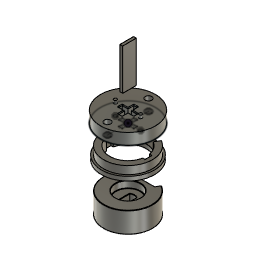
Zemismart Blinds.com Adapter (Autodesk Fusion 360 design; units mm, degrees)
Autodesk Fusion 360 part; units mm, degrees
sketch "Sketch1" plane through (0, 0, 0) normal (0, 0, 1) x (1, 0, 0) in component "Motor Driver"
  circle A0 centre (0, 0) radius 17.875
  line L0 (-9.0114, 15.4373) -> (8.9886, 15.4506)
  line L1 (-9.0114, 15.4373) -> (-5.0783, 15.4373) construction
  circle A1 centre (0, 0) radius 12.375 construction
  line L2 (-12.8986, 12.375) -> (12.8986, 12.375) construction
  line L3 (-9.0114, 15.4373) -> (-7.2434, 12.375)
  line L4 (-9.0114, 15.4373) -> (-5.4753, 15.4373) construction
  line L5 (8.9886, 15.4506) -> (7.2129, 12.375)
  line L6 (8.9886, 15.4506) -> (12.5579, 15.4506) construction
  line L7 (7.2129, 12.375) -> (-7.2434, 12.375)
  circle A2 centre (0, 0) radius 4.5
  line L8 (0, 0) -> (2.5, 0) construction
  line L9 (0, 0) -> (-2.5, 0) construction
  line L10 (-2.5, 0) -> (-2.5, 3.7417)
  line L11 (-2.5, 0) -> (-2.5, -3.7417)
  line L12 (2.5, 0) -> (2.5, -3.7417)
  line L13 (2.5, 0) -> (2.5, 3.7417)
  circle A3 centre (0, 0) radius 9.125
  dimension "d1" = 35.75
  dimension "d2" = 18
  dimension "d4" = 24.75
  dimension "d5" = 60
  dimension "d6" = 120
  dimension "d7" = 9
  dimension "d8" = 2.5
  dimension "d9" = 2.5
  dimension "d12" = 18.25
  constraint coincident A0.centre A1.centre
  constraint coincident A0 L0.start
  constraint coincident A0 L0.end
  constraint horizontal L1
  constraint coincident A0 L2.start
  constraint coincident A0 L2.end
  constraint horizontal L2
  constraint tangent A1 L2
  constraint horizontal L4
  constraint coincident L2 L3.end
  constraint horizontal L6
  constraint coincident L2 L5.end
  constraint concentric A1 A2
  constraint horizontal L8
  constraint parallel L8 L9
  constraint coincident A2 L10.end
  constraint perpendicular L9 L10
  constraint coincident A2 L11.end
  constraint perpendicular L9 L11
  constraint coincident A2 L12.end
  constraint perpendicular L8 L12
  constraint coincident A2 L13.end
  constraint perpendicular L8 L13
  constraint concentric A2 A3
  measures "d1" diameter of A0
  measures "d2" distance of L0.start L0.end
  measures "d4" diameter of A1
  measures "d5" angle of L3 L4
  measures "d6" angle of L5 L6
  measures "d7" diameter of A2
  measures "d8" distance of A0.centre L8.end
  measures "d9" distance of A0.centre L9.end
  measures "d12" diameter of A3
extrude "Extrude1" add sketch "Sketch1" along normal blind 15.25 contours A0 L3 L5 L7 | A2 L12 L13 | A2 L10 L11 | A3 makes body 1 in component "Motor Driver"
extrude "Extrude2" cut sketch "Sketch1" against normal blind 5 from surface at 15.25 contours A2 L12 L13 | A2 L10 L11 | A3 bodies 1 in component "Motor Driver"
fillet "Fillet1" radius 0.25 3 faces at (-4.7083, 0, 10.25) (9.1137, -0.4548, 11.9167) (9.0132, 10.2341, 15.25) on bodies 1 in component "Motor Driver"
fillet "Fillet2" radius 0.25 1 faces at (-0.0102, 9.75, 0) on bodies 1 in component "Motor Driver"
sketch "Sketch1 (2)" plane through (0, 0, 0) normal (0, 0, 1) x (1, 0, 0) in component "Motor Ring"
  circle A0 centre (0, 0) radius 17.875
  line L0 (-9.0114, 15.4373) -> (8.9886, 15.4506)
  line L1 (-9.0114, 15.4373) -> (-5.0783, 15.4373) construction
  circle A1 centre (0, 0) radius 2.5 construction
  line L2 (-17.6993, 2.5) -> (17.6993, 2.5) construction
  line L3 (-9.0114, 15.4373) -> (-1.5421, 2.5)
  line L4 (-9.0114, 15.4373) -> (-5.4753, 15.4373) construction
  line L5 (8.9886, 15.4506) -> (1.5115, 2.5)
  line L6 (8.9886, 15.4506) -> (12.5579, 15.4506) construction
  line L7 (1.5115, 2.5) -> (-1.5421, 2.5)
  dimension "d1_1" = 35.75
  dimension "d2_1" = 18
  dimension "d4_1" = 5
  dimension "d5_1" = 60
  dimension "d6_1" = 120
  constraint coincident A0.centre A1.centre
  constraint coincident A0 L0.start
  constraint coincident A0 L0.end
  constraint horizontal L1
  constraint coincident A0 L2.start
  constraint coincident A0 L2.end
  constraint horizontal L2
  constraint tangent A1 L2
  constraint horizontal L4
  constraint coincident L2 L3.end
  constraint horizontal L6
  constraint coincident L2 L5.end
  measures "d1_1" diameter of A0
  measures "d2_1" distance of L0.start L0.end
  measures "d4_1" diameter of A1
  measures "d5_1" angle of L3 L4
  measures "d6_1" angle of L5 L6
sketch "Ring Base" plane through (0, 0, 0) normal (0, 0, 1) x (1, 0, 0) in component "Motor Ring"
  circle A0 centre (0, 0) radius 19.375
  circle A1 centre (0, 0) radius 13.5
  line L0 (15, 2.5) -> (-15, 2.5)
  line L1 (-15, 2.5) -> (-15, -2.5)
  line L2 (-15, -2.5) -> (15, -2.5)
  line L3 (15, -2.5) -> (15, 2.5)
  line L4 (15, 2.5) -> (-15, -2.5) construction
  line L5 (-15, 2.5) -> (15, -2.5) construction
  dimension "d18" = 38.75
  dimension "d19" = 27
  dimension "d20" = 30
  dimension "d21" = 5
  constraint coincident A0.centre A1.centre
  constraint horizontal L0
  constraint perpendicular L0 L1
  constraint parallel L0 L2
  constraint parallel L1 L3
  constraint coincident L4 A0.centre
  constraint coincident L5 A0.centre
  measures "d18" diameter of A0
  measures "d19" diameter of A1
  measures "d20" distance of L1.end L2.end
  measures "d21" distance of L0.end L1.end
extrude "Extrude1'" add sketch "Ring Base" along normal blind 3 separate body makes body 2 in component "Motor Ring"
extrude "Extrude2'" add sketch "Sketch1 (2)" along normal blind 5.75 from surface at 3 contours A0 L3 L5 L7 bodies 2 in component "Motor Ring"
extrude "Extrude3" cut 1 faces at (9.3482, 0.8333, 3) along direction (0, 0, 1) blind 5.75 on bodies 2 bodies 2 in component "Motor Ring"
move_body "Move1" bodies 2 to x (1, 0, 0) y (0, 1, 0) z (0, 0, 1) at (0, 0, 25) in component "Motor Ring"
move_body "Move2" bodies 2 to x (1, 0, 0) y (0, 1, 0) z (0, 0, 1) at (0, 0, 10) in component "Motor Ring"
sketch "Sketch3" plane through (0, 0, 0) normal (0, 0, 1) x (1, 0, 0) in component "Motor Mount"
  line L0 (0, 0) -> (9.25, 0) construction
  circle A0 centre (9.25, 0) radius 1.125
  line L1 (0, 0) -> (-9.25, 0) construction
  circle A1 centre (-9.25, 0) radius 1.125
  dimension "d34_1" = 9.25
  dimension "d35_1" = 2.25
  dimension "d36_1" = 9.25
  dimension "d37_1" = 2.25
  constraint coincident L0.start L1.start
  constraint horizontal L0
  constraint coincident L0.end A0.centre
  constraint parallel L0 L1
  constraint coincident L1.end A1.centre
  measures "d34_1" distance of L0.start L0.end
  measures "d35_1" diameter of A0
  measures "d36_1" distance of L0.start L1.end
  measures "d37_1" diameter of A1
sketch "Sketch1 (3)" plane through (0, 0, 0) normal (0, 0, 1) x (1, 0, 0) in component "Motor Mount"
  circle A0 centre (0, 0) radius 20
  line L0 (0, 0) -> (0, 15) construction
  circle A1 centre (0, 15) radius 2.375
  line L1 (0, 0) -> (0, -15) construction
  circle A2 centre (0, -15) radius 2.375
  dimension "d1_2" = 40
  dimension "d2_2" = 15
  dimension "d3_1" = 4.75
  dimension "d4_2" = 15
  dimension "d5_2" = 4.75
  constraint coincident A0.centre L0.start
  constraint vertical L0
  constraint coincident L0.end A1.centre
  constraint vertical L1
  constraint coincident L1.end A2.centre
  measures "d1_2" diameter of A0
  measures "d2_2" distance of A0.centre L0.end
  measures "d3_1" diameter of A1
  measures "d4_2" distance of A0.centre L1.end
  measures "d5_2" diameter of A2
extrude "Extrude1''" add sketch "Sketch1 (3)" along normal blind 8.25 separate body makes body 3 in component "Motor Mount"
sketch "Sketch2" plane through (0, 0, 0) normal (0, 0, 1) x (1, 0, 0) in component "Motor Mount"
  line L0 (5.5, 1.25) -> (-5.5, 1.25)
  line L1 (-5.5, 1.25) -> (-5.5, -1.25)
  line L2 (-5.5, -1.25) -> (5.5, -1.25)
  line L3 (5.5, -1.25) -> (5.5, 1.25)
  line L4 (5.5, 1.25) -> (-5.5, -1.25) construction
  line L5 (-5.5, 1.25) -> (5.5, -1.25) construction
  line L6 (1.25, 5.5) -> (-1.25, 5.5)
  line L7 (-1.25, 5.5) -> (-1.25, -5.5)
  line L8 (-1.25, -5.5) -> (1.25, -5.5)
  line L9 (1.25, -5.5) -> (1.25, 5.5)
  line L10 (1.25, 5.5) -> (-1.25, -5.5) construction
  line L11 (-1.25, 5.5) -> (1.25, -5.5) construction
  dimension "d46_1" = 11
  dimension "d47_1" = 2.5
  dimension "d52_1" = 2.5
  dimension "d53_1" = 11
  constraint horizontal L0
  constraint perpendicular L0 L1
  constraint parallel L0 L2
  constraint parallel L1 L3
  constraint coincident L4 origin
  constraint coincident L5 origin
  constraint horizontal L6
  constraint perpendicular L6 L7
  constraint parallel L6 L8
  constraint parallel L7 L9
  constraint coincident L10 origin
  constraint coincident L11 origin
  measures "d46_1" distance of L1.end L2.end
  measures "d47_1" distance of L0.end L1.end
  measures "d52_1" distance of L7.end L8.end
  measures "d53_1" distance of L6.end L7.end
extrude "Extrude3'" add sketch "Sketch3" along normal blind 2.25 from surface at 8.25 bodies 3 in component "Motor Mount"
chamfer "Chamfer1" distance 0.75 angle 45 1 edges at (-2.2143, -14.1412, 0) on bodies 3 in component "Motor Mount"
chamfer "Chamfer2" distance 0.75 angle 45 1 edges at (-2.2143, 15.8588, 0) on bodies 3 in component "Motor Mount"
extrude "Extrude4" cut sketch "Sketch2" against normal blind 8 from surface at 8.25 bodies 3 in component "Motor Mount"
fillet "Fillet3" radius 0.5 6 edges at (3.375, 1.25, 8.25) (-3.375, 1.25, 8.25) (-5.5, 0, 8.25) (3.375, -1.25, 8.25) (-3.375, -1.25, 8.25) (5.5, 0, 8.25) on bodies 3 in component "Motor Mount"
fillet "Fillet3" radius 0.5 6 edges at (-1.25, 3.375, 8.25) (0, 5.5, 8.25) (1.25, 3.375, 8.25) (1.25, -3.375, 8.25) (0, -5.5, 8.25) (-1.25, -3.375, 8.25) on bodies 3 in component "Motor Mount"
copy_body "CutPasteBodies1" bodies 3 removing the originals makes body 4 in component "Motor Mount"
sketch "Sketch4" plane through (0, 0, 0) normal (0, 0, 1) x (1, 0, 0) in component "Insert"
  line L0 (27.8064, -0.0636) -> (57.8064, -0.0636)
  line L1 (57.8064, -0.0636) -> (57.8064, 9.9364)
  line L2 (57.8064, 9.9364) -> (27.8064, 9.9364)
  line L3 (27.8064, 9.9364) -> (27.8064, -0.0636)
  dimension "d55_1" = 30
  dimension "d56_1" = 10
  constraint horizontal L0
  constraint vertical L1
  constraint horizontal L2
  constraint vertical L3
  measures "d55_1" distance of L0.start L0.end
  measures "d56_1" distance of L0.start L2.end
extrude "Extrude5" add sketch "Sketch4" along normal blind 2 separate body makes body 5 in component "Insert"
copy_body "CutPasteBodies1'" bodies 5 removing the originals makes body 6 in component "Insert"
move_body "Move1'" bodies 6 to x (1, 0, 0) y (0, 1, 0) z (0, 0, 1) at (-3.2429, 19.9544, 23.1973) in component "Insert"
move_body "Move2'" bodies 6 to x (0, 0, -1) y (0, 1, 0) z (1, 0, 0) at (31.3662, 0, 77.7608) in component "Insert"
move_body "Move3" bodies 6 to x (1, 0, 0) y (0, 1, 0) z (0, 0, 1) at (-55.5746, -36.7232, 2.0622) in component "Insert"
move_body "Move4" bodies 6 to x (1, 0, 0) y (0, 1, 0) z (0, 0, 1) at (0, 11.9024, -5.3753) in component "Insert"
component "Motor Driver" placed x (1, 0, 0) y (0, 1, 0) z (0, 0, 1) at (0, 0, 0)
component "Motor Ring" placed x (1, 0, 0) y (0, 1, 0) z (0, 0, 1) at (0, 0, 0)
component "Motor Mount" placed x (1, 0, 0) y (0, 1, 0) z (0, 0, 1) at (0, 0, 0)
component "Insert" placed x (1, 0, 0) y (0, 1, 0) z (0, 0, 1) at (0, 0, 0)
equation "d6_2 = 18.25 mm - 10 mm"
equation "d53_1 = d46_1"
named bodies: "Motor Driver", "Motor Ring", "Motor Mount", "Insert"
